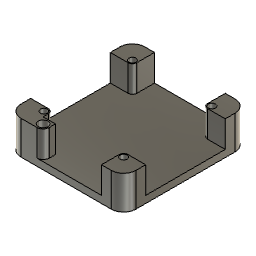
orangeBoxUp_2 (Autodesk Fusion 360 design; units mm, degrees)
Autodesk Fusion 360 part; units mm, degrees
note: some values were not read from the file. Chosen so that the rebuilt part matches the saved one: which face or edge a step refers to; which pieces of a blend or face edit are solid. Set by a fixed rule: which sketch regions a step uses.
sketch "Sketch1" plane through (0, 0, 0) normal (0, 0, 1) x (1, 0, 0)
  line L0 (0, 0) -> (60, 0)
  line L1 (60, 0) -> (60, 60)
  line L2 (60, 60) -> (0, 60)
  line L3 (0, 60) -> (0, 0)
  line L4 (2, 2) -> (58, 2)
  line L5 (58, 2) -> (58, 58)
  line L6 (58, 58) -> (2, 58)
  line L7 (2, 58) -> (2, 2)
  dimension "d1" = 60
  dimension "d2" = 60
  dimension "d3" = 56
  dimension "d4" = 56
  constraint horizontal L0
  constraint vertical L1
  constraint horizontal L2
  constraint vertical L3
  constraint coincident L0.start L3.end
  constraint horizontal L4
  constraint vertical L5
  constraint horizontal L6
  constraint vertical L7
  measures "d1" distance of L0.start L0.end
  measures "d2" distance of L0.start L2.end
  measures "d3" distance of L4.start L4.end
  measures "d4" distance of L4.start L6.end
sketch "Sketch2" plane through (0, 0, 2) normal (0, 0, 1) x (-1, 0, 0)
  line L0 (-2, -2) -> (-4.5, -2)
  line L1 (-4.5, -2) -> (-4.5, -5)
  line L2 (-4.5, -5) -> (-2, -5)
  line L3 (-2, -5) -> (-2, -2)
  line L4 (-2, -58) -> (-4.5, -58)
  line L5 (-4.5, -58) -> (-4.5, -55)
  line L6 (-4.5, -55) -> (-2, -55)
  line L7 (-2, -55) -> (-2, -58)
  line L8 (-58, -58) -> (-49.5, -58)
  line L9 (-49.5, -58) -> (-49.5, -55)
  line L10 (-49.5, -55) -> (-58, -55)
  line L11 (-58, -55) -> (-58, -58)
  line L12 (-58, -2) -> (-49.5, -2)
  line L13 (-49.5, -2) -> (-49.5, -5)
  line L14 (-49.5, -5) -> (-58, -5)
  line L15 (-58, -5) -> (-58, -2)
  circle A0 centre (-4.5, -55) radius 1
  circle A1 centre (-49.5, -55) radius 1
  circle A2 centre (-4.5, -5) radius 1
  circle A3 centre (-49.5, -5) radius 1
  line L16 (-2, -58) -> (-2, -2)
  line L17 (-2, -2) -> (-58, -2)
  line L18 (-58, -2) -> (-58, -58)
  line L19 (-58, -58) -> (-2, -58)
  dimension "d9" = 2.5
  dimension "d10" = 3
  dimension "d11" = 2.5
  dimension "d12" = 3
  dimension "d13" = 8.5
  dimension "d14" = 3
  dimension "d15" = 8.5
  dimension "d16" = 3
  dimension "d17" = 2
  dimension "d18" = 2
  dimension "d19" = 2
  dimension "d20" = 2
  constraint horizontal L0
  constraint vertical L1
  constraint horizontal L2
  constraint vertical L3
  constraint horizontal L4
  constraint vertical L5
  constraint horizontal L6
  constraint vertical L7
  constraint horizontal L8
  constraint vertical L9
  constraint horizontal L10
  constraint vertical L11
  constraint horizontal L12
  constraint vertical L13
  constraint horizontal L14
  constraint vertical L15
  constraint coincident L5.end L6.start
  constraint coincident L9.end L10.start
  constraint coincident L1.end L2.start
  constraint coincident L13.end L14.start
  measures "d9" distance of L0.start L0.end
  measures "d10" distance of L0.start L2.end
  measures "d11" distance of L4.start L4.end
  measures "d12" distance of L4.start L6.end
  measures "d13" distance of L8.start L8.end
  measures "d14" distance of L8.start L10.end
  measures "d15" distance of L12.start L12.end
  measures "d16" distance of L12.start L14.end
  measures "d17" diameter of A0
  measures "d18" diameter of A1
  measures "d19" diameter of A2
  measures "d20" diameter of A3
sketch "Sketch3" plane through (0, 0, 0) normal (0, 0, 1) x (1, 0, 0)
  circle A0 centre (0, 45) radius 2
  circle A1 centre (50, 45) radius 2
  circle A2 centre (50, 0) radius 2
  circle A3 centre (0, 0) radius 2
  line L0 (0, -2.5) -> (50, -2.5)
  line L1 (52.5, 0) -> (52.5, 45)
  line L2 (-2.5, 0.0027) -> (-2.5, 45)
  line L3 (0.0001, 47.5) -> (50, 47.5)
  circle A4 centre (0, 45) radius 7.5
  circle A5 centre (0, 0) radius 7.5
  circle A6 centre (50, 45) radius 7.5
  circle A7 centre (50, 0) radius 7.5
  line L4 (0, 42.5) -> (-7.0711, 42.5)
  line L5 (2.5, 45) -> (2.5, 52.0711)
  line L6 (47.5, 45) -> (47.5, 52.0711)
  line L7 (50, 42.5) -> (57.0711, 42.5)
  line L8 (50, 2.5) -> (57.0711, 2.5)
  line L9 (47.5, 0) -> (47.5, -7.0711)
  line L10 (0, 2.5) -> (-7.0711, 2.5)
  line L11 (2.5, 0) -> (2.5, -7.0711)
  arc A8 (0, 42.5) -> (2.5, 45) centre (0, 45) ccw
  arc A9 (0.0001, 47.5) -> (-2.5, 45) centre (0, 45) ccw
  line L12 (0, 45) -> (0, 43)
  line L13 (2, 45) -> (0, 45)
  arc A10 (47.5, 45) -> (50, 42.5) centre (50, 45) ccw
  arc A11 (52.5, 45) -> (50, 47.5) centre (50, 45) ccw
  line L14 (50, 43) -> (50, 45)
  line L15 (50, 45) -> (48, 45)
  line L16 (47.5, 45) -> (2.5, 45)
  arc A12 (50, 2.5) -> (47.5, 0) centre (50, 0) ccw
  arc A13 (50, -2.5) -> (52.5, 0) centre (50, 0) ccw
  line L17 (48, 0) -> (50, 0)
  line L18 (50, 0) -> (50, 2)
  line L19 (50, 2.5) -> (50, 42.5)
  arc A14 (-2.5, 0.0027) -> (0, -2.5) centre (0, 0) ccw
  arc A15 (2.5, 0) -> (0, 2.5) centre (0, 0) ccw
  line L20 (0, 0) -> (2, 0)
  line L21 (2.5, 0) -> (47.5, 0)
  line L22 (0, 42.5) -> (0, 2.5)
  line L23 (0, 2) -> (0, 0)
  dimension "d23" = 50
  dimension "d24" = 45
  dimension "d25" = 4
  dimension "d26" = 4
  dimension "d27" = 4
  dimension "d28" = 4
  dimension "d29" = 5
  dimension "d30" = 5
  dimension "d31" = 5
  dimension "d32" = 5
  dimension "d37" = 15
  dimension "d38" = 15
  dimension "d39" = 15
  dimension "d40" = 15
  constraint horizontal L20
  constraint vertical L18
  constraint horizontal L15
  constraint vertical L12
  constraint coincident A3.centre A5.centre
  constraint coincident A0.centre A4.centre
  constraint coincident A1.centre A6.centre
  constraint coincident A2.centre A7.centre
  constraint concentric A0 A8
  constraint concentric A1 A10
  constraint concentric A2 A12
  constraint coincident L0.end A12
  constraint tangent L0 A12
  constraint perpendicular L0 L12
  constraint coincident L1.end A10
  constraint tangent L1 A10
  constraint perpendicular L0 L1
  constraint tangent L2 A8
  constraint coincident L3.start A8
  constraint tangent L3 A10
  constraint concentric A0 A4
  constraint concentric A1 A6
  constraint concentric A7 A12
  constraint coincident L4.start L12
  constraint coincident A4 L4.end
  constraint tangent L4 A8
  constraint coincident A4 L5.end
  constraint tangent L5 A8
  constraint coincident L6.start L15
  constraint coincident A6 L6.end
  constraint tangent L6 A10
  constraint perpendicular L3 L6
  constraint coincident A6 L7.end
  constraint tangent L7 A10
  constraint coincident L8.start L18
  constraint coincident A7 L8.end
  constraint tangent L8 A12
  constraint coincident A7 L9.end
  constraint tangent L9 A12
  constraint coincident L10.start L12
  constraint coincident A5 L10.end
  constraint tangent L10 A14
  constraint coincident L11.start A14
  constraint coincident L11.start L20
  constraint coincident A5 L11.end
  constraint tangent L11 A14
  constraint concentric A8 A9
  constraint coincident A0 L12.end
  constraint collinear L12 L22
  constraint coincident A0 L13.start
  constraint collinear L13 L15
  constraint concentric A10 A11
  constraint coincident A1 L14.start
  constraint collinear L14 L18
  constraint coincident A1 L15.end
  constraint collinear L15 L16
  constraint concentric A12 A13
  constraint coincident A2 L17.start
  constraint collinear L17 L20
  constraint coincident A2 L18.end
  constraint collinear L18 L19
  constraint concentric A14 A15
  constraint coincident A3 L20.end
  constraint collinear L20 L21
  constraint coincident A3 L23.start
  constraint collinear L22 L23
  measures "d23" distance of A3.centre A2.centre
  measures "d24" distance of A3.centre A0.centre
  measures "d25" diameter of A0
  measures "d26" diameter of A1
  measures "d27" diameter of A2
  measures "d28" diameter of A3
  measures "d29" diameter of A14
  measures "d30" diameter of A8
  measures "d31" diameter of A10
  measures "d32" diameter of A12
  measures "d37" diameter of A4
  measures "d38" diameter of A5
  measures "d39" diameter of A6
  measures "d40" diameter of A7
extrude "Extrude6" add sketch "Sketch3" along normal blind 7 contours L0 L2 A5 L10 L11 A14 | L0 L1 A7 L8 L9 A13 | L2 L3 A4 L4 L5 A9 | L1 L3 A6 L6 L7 A11 makes body 1 at (48.1731, 52.2741, 2.3333) makes body 2 at (48.8622, -7.4132, 4.6667) makes body 3 at (-7.4132, 43.8622, 2.3333) makes body 4 at (2.1658, -7.1805, 4.6667)
extrude "Extrude7" add sketch "Sketch3" along normal blind 2 separate body contours L0 A5 L11 L21 | L0 A5 A7 L21 | A5 A15 L21 L22 | L2 A5 L10 L22 | L0 A7 L9 L21 | A4 A5 A6 A7 L16 L19 L21 L22 | L2 A4 A5 L22 | A7 A12 L19 L21 | L2 A4 L4 L22 | L1 A6 A7 L19 | L1 A7 L8 L19 | A4 A8 L16 L22 | L1 A6 L7 L19 | A6 A10 L16 L19 | L3 A4 L5 L16 | L3 A4 A6 L16 | L3 A6 L6 L16 makes body 5
extrude "Extrude8" add sketch "Sketch3" along normal blind 6 contours L0 L2 L10 L11 A14 A15 | L0 L1 L8 L9 A12 A13 | L2 L3 L4 L5 A8 A9 | L1 L3 L6 L7 A10 A11 bodies 1 2 3 4 5
sketch "Sketch4" plane through (0, 0, 7) normal (0, 0, 1) x (-1, 0, 0)
  line L0 (-2.5, -47.5) -> (-2.5, -52.0711)
  arc A0 (-2.5, -52.0711) -> (7.0711, -42.5) centre (0, -45) ccw
  line L1 (7.0711, -42.5) -> (2.5, -42.5)
  line L2 (2.5, -42.5) -> (2.5, -45)
  arc A1 (-0.0001, -47.5) -> (2.5, -45) centre (0, -45) ccw
  line L3 (-0.0001, -47.5) -> (-2.5, -47.5)
  line L4 (3.0524, -42.5) -> (-2.4476, -42.5)
  line L5 (-2.4476, -42.5) -> (-2.4476, -48)
  line L6 (-2.4476, -48) -> (3.0524, -48)
  line L7 (3.0524, -48) -> (3.0524, -42.5)
  line L8 (-53.0435, -42.4424) -> (-47.5435, -42.4424)
  line L9 (-47.5435, -42.4424) -> (-47.5435, -47.9424)
  line L10 (-47.5435, -47.9424) -> (-53.0435, -47.9424)
  line L11 (-53.0435, -47.9424) -> (-53.0435, -42.4424)
  line L12 (-47, 3) -> (-53, 3)
  line L13 (-53, 3) -> (-53, -3)
  line L14 (-53, -3) -> (-47, -3)
  line L15 (-47, -3) -> (-47, 3)
  line L16 (-3, 3) -> (3, 3)
  line L17 (3, 3) -> (3, -3)
  line L18 (3, -3) -> (-3, -3)
  line L19 (-3, -3) -> (-3, 3)
  dimension "d47" = 5.5
  dimension "d48" = 5.5
  dimension "d49" = 5.5
  dimension "d50" = 5.5
  constraint horizontal L4
  constraint vertical L5
  constraint horizontal L6
  constraint vertical L7
  constraint coincident L1 L4.start
  constraint horizontal L8
  constraint vertical L9
  constraint horizontal L10
  constraint vertical L11
  constraint horizontal L12
  constraint vertical L13
  constraint horizontal L14
  constraint vertical L15
  constraint horizontal L16
  constraint vertical L17
  constraint horizontal L18
  constraint vertical L19
  measures "d47" distance of L4.start L4.end
  measures "d48" distance of L4.start L6.end
  measures "d49" distance of L8.start L8.end
  measures "d50" distance of L8.start L10.end
extrude "Extrude9" cut sketch "Sketch4" against normal blind 1 contours L1 L2 A1 L3 L4 L5 L6 L7 | L8 L9 L10 L11 | L12 L13 L14 L15 | L16 L17 L18 L19 bodies 1
extrude "Extrude10" cut 4 faces at (52.6956, 45.1475, 6) (-2.7016, 45.1667, 6) (-0.1168, -2.6648, 6) (50.2165, -2.6648, 6) along direction (0, 0, -1) blind 1 on bodies 1 bodies 1
extrude "Extrude11" cut 4 faces at (50.4007, 49.4532, 7) (50.3718, -4.4916, 7) (-4.4916, -0.3718, 7) (-0.4067, 49.4916, 7) along direction (0, 0, -1) blind 1 on bodies 1 bodies 1
extrude "Extrude12" add 4 faces at (-4.4916, -0.3718, 6) (-0.4067, 49.4916, 6) (50.4007, 49.4532, 6) (50.3718, -4.4916, 6) along direction (0, 0, 1) blind 0.5 on bodies 1 bodies 1
delete_face "DeleteFace1" 2 faces at (2.4651, 47.5, 5.5) (2.4476, 47.6667, 6) on bodies 1
sketch "Sketch5" plane through (0, 0, 0) normal (0, 0, -1) x (1, 0, 0)
  line L0 (-2.5, -2.5) -> (-2.5, -42.5)
  line L1 (-2.5, -42.5) -> (-7.0711, -42.5)
  arc A0 (-7.0711, -42.5) -> (2.5, -52.0711) centre (0, -45) ccw
  line L2 (2.5, -52.0711) -> (2.5, -47.5)
  line L3 (2.5, -47.5) -> (47.5, -47.5)
  line L4 (47.5, -47.5) -> (47.5, -52.0711)
  arc A1 (47.5, -52.0711) -> (57.0711, -42.5) centre (50, -45) ccw
  line L5 (57.0711, -42.5) -> (52.5, -42.5)
  line L6 (52.5, -42.5) -> (52.5, -2.5)
  line L7 (52.5, -2.5) -> (57.0711, -2.5)
  arc A2 (57.0711, -2.5) -> (47.5, 7.0711) centre (50, 0) ccw
  line L8 (47.5, 7.0711) -> (47.5, 2.5)
  line L9 (47.5, 2.5) -> (2.5, 2.5)
  line L10 (2.5, 2.5) -> (2.5, 7.0711)
  arc A3 (2.5, 7.0711) -> (-7.0711, -2.5) centre (0, 0) ccw
  line L11 (-7.0711, -2.5) -> (-2.5, -2.5)
  circle A4 centre (0, 0) radius 2
  circle A5 centre (50, -45) radius 2
  circle A6 centre (0, -45) radius 2
  circle A7 centre (50, 0) radius 2
  circle A8 centre (-5.25, -39.75) radius 2.75
  circle A9 centre (-5.25, -39.75) radius 3.8891
  circle A10 centre (-5.25, -39.75) radius 2
  line L12 (-3.5001, -38.7816) -> (-2.5, -38.7816)
  line L13 (-3.5001, -40.7184) -> (-2.5, -40.7184)
  line L14 (-7.0711, -42.5) -> (-7.0711, -41.8106)
  dimension "d59" = 2.75
  dimension "d61" = 4
  constraint tangent L1 A8
  constraint tangent L0 A8
  constraint concentric A8 A9
  constraint coincident L0.end A9
  constraint concentric A9 A10
  constraint coincident A10 L12.start
  constraint coincident L0 L12.end
  constraint perpendicular L0 L12
  constraint coincident A10 L13.start
  constraint coincident L0 L13.end
  constraint perpendicular L0 L13
  constraint coincident L1.end A0.start
  constraint coincident A8 L14.end
  constraint perpendicular L1 L14
  measures "d59" radius of A8
  measures "d61" diameter of A10
extrude "Extrude13" add sketch "Sketch5" against normal blind 16 contours L0 A0 A8 A9 L12 L14 | L0 A8 L12 | L1 A8 L14 bodies 1
delete_face "DeleteFace2" 1 faces at (-7.5685, 42.8725, 7.5) on bodies 1
delete_face "DeleteFace3" 1 faces at (-2.5096, 39.5203, 6) on bodies 1
delete_face "DeleteFace4" 1 faces at (-5.4797, 42.4904, 7.5) on bodies 1
extrude "Extrude14" add sketch "Sketch5" against normal blind 16 contours L0 A0 A8 A9 L12 L14 bodies 1
extrude "Extrude15" add sketch "Sketch5" against normal blind 9 contours A8 A10 L12 L13 | L0 L1 A8 L13 | L1 A8 L14 picked at (-7.0528, -41.4744) bodies 1
extrude "Extrude16" add sketch "Sketch5" against normal blind 2 contours L0 A8 L12 | A8 A10 L12 L13 | L0 A8 L13 | A8 A10 L12 L13 | A10 bodies 1
fillet "Fillet1" radius 1 1 edges at (-2.5, 38.7816, 9) on bodies 1
fillet "Fillet2" radius 1 1 edges at (-2.5, 40.7184, 5.5) on bodies 1
extrude "Extrude17" add 1 faces at (-7.425, 42.2236, 16) along direction (0, 0, 1) blind 7.5 on bodies 1 bodies 1
sketch "Sketch6" plane through (0, 0, 0) normal (0, 0, 1) x (1, 0, 0)
sketch "Sketch7" plane through (0, 0, 0) normal (0, 0, 1) x (1, 0, 0)
  line L0 (0, -56) -> (-3, -56)
  line L1 (-3, -56) -> (-3, -53)
  line L2 (-3, -53) -> (0, -53)
  line L3 (0, -53) -> (0, -56)
  line L4 (-51, -56) -> (-48, -56)
  line L5 (-51, -53) -> (-51, -56)
  circle A0 centre (-3, -53) radius 2
  circle A1 centre (-48, -53) radius 2
  circle A2 centre (-3, -3) radius 2
  circle A3 centre (-48, -3) radius 2
  circle A4 centre (-3, -3) radius 2.5
  circle A5 centre (-3, -53) radius 2.5
  circle A6 centre (-48, -53) radius 2.5
  circle A7 centre (-48, -3) radius 2.5
  line L6 (-45.5, -3) -> (-45.5, 0)
  line L7 (-48, -5.5) -> (-51, -5.5)
  line L8 (-48, -50.5) -> (-51, -50.5)
  line L9 (-45.5, -52.9982) -> (-45.4978, -56)
  line L10 (-5.5, -52.9982) -> (-5.5022, -56)
  line L11 (-3, -50.5) -> (0, -50.5)
  line L12 (-3, -5.5) -> (0, -5.5)
  line L13 (-5.5, -3) -> (-5.5, 0)
  line L14 (7, -56) -> (7, 0)
  line L15 (0, 7) -> (-51, 7)
  line L16 (-58, 0) -> (-58, -56)
  line L17 (-51, -63) -> (0, -63)
  line L18 (-5.5022, -56) -> (-5.5022, -63)
  line L19 (0, -50.5) -> (7, -50.5)
  line L20 (0, -5.5) -> (7, -5.5)
  line L21 (-51, -5.5) -> (-58, -5.5)
  line L22 (-45.5, 0) -> (-45.5, 7)
  line L23 (-5.5, 0) -> (-5.5, 7)
  arc A8 (7, 0) -> (0, 7) centre (0, 0) ccw
  line L24 (0, 0) -> (-5.5, 0)
  line L25 (-44, 0) -> (-51, 0)
  arc A9 (0, -63) -> (7, -55.9966) centre (0, -56) ccw
  line L26 (0, -56) -> (0, -50.5)
  line L27 (0, -5.5) -> (0, 0)
  line L28 (-45.4978, -56) -> (-45.4978, -63)
  line L29 (-51, -50.5) -> (-58, -50.5)
  arc A10 (-58, -56) -> (-51, -63) centre (-51, -56) ccw
  line L30 (-51, 0) -> (-51, -7)
  line L31 (-51, -50.5) -> (-51, -56)
  arc A11 (-51, 7) -> (-58, 0) centre (-51, 0) ccw
  line L32 (-51, -56) -> (-45.4978, -56)
  line L33 (-5.5022, -56) -> (0, -56)
  line L34 (-5.5022, -56) -> (-45.4978, -56)
  circle A12 centre (-41.9978, -59.5) radius 2.75
  circle A13 centre (-41.9978, -59.5) radius 2
  line L35 (-38.4978, -59.5016) -> (-38.4962, -56)
  arc A14 (-41.9978, -63) -> (-38.4978, -59.5016) centre (-41.9978, -59.5) ccw
  line L36 (-43, -56) -> (-43, -57.7692)
  line L37 (-41, -56) -> (-41, -57.7667)
  dimension "d76" = 51
  dimension "d77" = 56
  dimension "d78" = 3
  dimension "d79" = 3
  dimension "d82" = 4
  dimension "d83" = 4
  dimension "d84" = 4
  dimension "d85" = 4
  dimension "d86" = 5
  dimension "d87" = 5
  dimension "d88" = 5
  dimension "d89" = 5
  dimension "d90" = 14
  dimension "d91" = 14
  dimension "d92" = 14
  dimension "d93" = 14
  dimension "d101" = 3.5
  dimension "d102" = 5.5
  dimension "d103" = 4
  constraint horizontal L24
  constraint vertical L30
  constraint horizontal L32
  constraint vertical L26
  constraint coincident A8.centre L24.start
  constraint horizontal L0
  constraint vertical L1
  constraint horizontal L2
  constraint vertical L3
  constraint horizontal L4
  constraint vertical L5
  constraint coincident L1.end L2.start
  constraint concentric A2 A4
  constraint concentric A0 A5
  constraint concentric A1 A6
  constraint concentric A3 A7
  constraint coincident A7 L6.start
  constraint coincident L6.end L24
  constraint perpendicular L6 L24
  constraint coincident A7 L7.start
  constraint coincident L7.end L30
  constraint perpendicular L7 L30
  constraint coincident A6 L8.start
  constraint coincident L8.end L30
  constraint tangent A6 L8
  constraint coincident A6 L9.start
  constraint tangent A6 L9
  constraint coincident A5 L10.start
  constraint coincident L10.end L32
  constraint tangent A5 L10
  constraint coincident A5 L11.start
  constraint perpendicular L11 L26
  constraint coincident A4 L12.start
  constraint coincident L12.end L26
  constraint perpendicular L12 L26
  constraint coincident A4 L13.start
  constraint perpendicular L13 L24
  constraint coincident L0.start L3.end
  constraint coincident L25.end L30.start
  constraint coincident L4.start L5.end
  constraint coincident L14.start A9
  constraint tangent L14 A8
  constraint tangent L15 A11
  constraint tangent L16 A10
  constraint tangent L17 A9
  constraint coincident L17 L18.end
  constraint perpendicular L17 L18
  constraint coincident L14 L19.end
  constraint perpendicular L14 L19
  constraint coincident L14 L20.end
  constraint perpendicular L14 L20
  constraint coincident L16 L21.end
  constraint perpendicular L16 L21
  constraint coincident L15 L22.end
  constraint perpendicular L15 L22
  constraint coincident L15 L23.end
  constraint perpendicular L15 L23
  constraint collinear L24 L25
  constraint coincident L14 A9.end
  constraint collinear L26 L27
  constraint coincident L17 L28.end
  constraint perpendicular L17 L28
  constraint coincident L16 L29.end
  constraint perpendicular L16 L29
  constraint collinear L30 L31
  constraint collinear L32 L33
  constraint tangent L34 A14
  constraint tangent L28 A14
  constraint concentric A12 A14
  constraint concentric A13 A14
  constraint coincident L34 L35.end
  constraint tangent L35 A14
  constraint coincident L17 A14.start
  constraint coincident L34 L36.start
  constraint coincident A13 L36.end
  constraint perpendicular L34 L36
  constraint coincident L34 L37.start
  constraint coincident A13 L37.end
  constraint perpendicular L34 L37
  measures "d76" distance of A8.centre L25.end
  measures "d77" distance of A8.centre L0.start
  measures "d78" distance of L0.start L0.end
  measures "d79" distance of L0.start L2.end
  measures "d82" diameter of A0
  measures "d83" diameter of A1
  measures "d84" diameter of A2
  measures "d85" diameter of A3
  measures "d86" diameter of A4
  measures "d87" diameter of A5
  measures "d88" diameter of A6
  measures "d89" diameter of A7
  measures "d90" diameter of A9
  measures "d91" diameter of A8
  measures "d92" diameter of A11
  measures "d93" diameter of A10
  measures "d101" radius of A14
  measures "d102" diameter of A12
  measures "d103" diameter of A13
extrude "Extrude18" add sketch "Sketch7" along normal blind 4 separate body contours A4 A5 A6 A7 L6 L7 L8 L9 L10 L11 L12 L13 L14 L15 L16 L19 L20 L21 L22 L23 L29 L34 | L17 L18 L34 L35 A14 | L17 L28 L34 A12 L35 A14 L36 L37 | L34 A12 L36 L37 | A12 A13 L36 L37 | A12 A13 L36 L37 | A13 makes body 6
extrude "Extrude19" add sketch "Sketch7" along normal blind 8.5 contours L0 L3 L14 L17 L18 L19 A9 L26 L33 | L14 L15 L20 L23 A8 L24 L27 | L4 L5 L16 L17 L28 L29 A10 L31 L32 | L15 L16 L21 L22 L25 L30 A11 bodies 6
extrude "Extrude20" add sketch "Sketch7" along normal blind 7 contours L0 L1 L2 L3 A5 L26 L33 | L1 A5 L10 L33 | L2 A5 L11 L26 | L1 L2 A0 A5 | L1 L2 A0 A5 | A4 L12 L13 L24 L27 | L4 L5 A6 L8 L9 L31 L32 | A4 | A6 | A7 L6 L7 L25 L30 | A7 bodies 6
extrude "Extrude21" cut sketch "Sketch7" along normal blind 10 contours L17 L28 L34 A12 L35 A14 L36 L37 | A12 A13 L36 L37 picked at (-40.6386, -57.4095) bodies 6
extrude "Extrude22" add sketch "Sketch7" along normal blind 8.5 contours L17 L28 L34 A12 L35 A14 L36 L37 | A12 A13 L36 L37 picked at (-40.6386, -57.4095) bodies 6
extrude "Extrude23" add 3 faces at (-1.7231, -55.6064, 7) (-2.8832, -0.3352, 7) (-50.6006, -54.2893, 7) along direction (0, 0, 1) blind 1.5 on bodies 6 bodies 6
extrude "Extrude24" cut sketch "Sketch7" along normal blind 10 contours A12 A13 L36 L37 | A12 A13 L36 L37 | A13 bodies 6
extrude "Extrude25" cut sketch "Sketch7" along normal blind 10 contours L34 A12 L36 L37 bodies 6
extrude "Extrude26" add sketch "Sketch7" along normal blind 8.5 contours L34 A12 L36 L37 bodies 6
extrude "Extrude27" add 1 faces at (-48.2165, -0.3352, 7) along direction (0, 0, 1) blind 1.5 on bodies 6 bodies 6
extrude "Extrude28" add 10 faces at (-48.2165, -0.3352, 8.5) (-53.3333, -1.8333, 8.5) (4.6667, -3.6667, 8.5) (-2.8341, -60.6667, 8.5) (-44.0694, -56.4495, 8.5) (-41.9319, -56.2525, 8.5) (-48.1659, -60.6667, 8.5) (-2.8832, -0.3352, 8.5) (-1.7231, -55.6064, 8.5) (-50.6006, -54.2893, 8.5) along direction (0, 0, 1) blind 10.5 on bodies 6 bodies 6
hidden bodies 1
